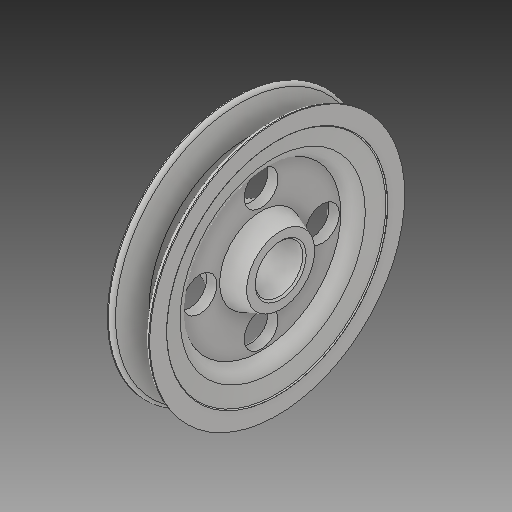
# Autodesk Inventor part: kladka
Saved by Autodesk Inventor 2019 (Build 230136000, 136)
## iProperties
Created: 2018-11-24
Part Number: kladka
Material: Generic
Document SubType Name: Modeling
Designer: Radek
Density: 1 g/cm^3
Appearance: Default
Author: Radek
Autodesk Inventor part; units mm, degrees
ref_plane "YZ Plane" through (0, 0, 0) normal (1, 0, 0) x (0, 1, 0)
ref_plane "XZ Plane" through (0, 0, 0) normal (0, 1, 0) x (-1, 0, 0)
ref_plane "XY Plane" through (0, 0, 0) normal (0, 0, 1) x (1, 0, 0)
sketch "Náčrt1" plane through (0, 0, 0) normal (0, 1, 0) x (-1, 0, 0)
  line L0 (14.5, -14) -> (-14.5, -14)
  line L1 (-14.5, -14) -> (-14.5, -20)
  line L2 (-14.5, -20) -> (-3, -24.4144)
  line L3 (-3, -24.4144) -> (-3, -46.8905)
  line L4 (14.5, -14) -> (14.5, -20)
  line L5 (14.5, -20) -> (3, -24.4144)
  line L6 (3, -24.4144) -> (3, -46.8905)
  line L7 (0, 0) -> (-43.8955, 0)
  line L8 (0, -90.4918) -> (0, 15.082) projected
  line L9 (-12.5, -75) -> (-12.5, -65)
  line L10 (12.5, -75) -> (12.5, -65)
  arc A0 (5.3126, -57.5064) -> (-5.3126, -57.5064) centre (0, -58.9299) ccw
  line L11 (-12.5, -75) -> (-11.9183, -75)
  line L12 (-9.5035, -73.147) -> (-5.3126, -57.5064)
  arc A1 (-11.9183, -75) -> (-9.5035, -73.147) centre (-11.9183, -72.5) ccw
  line L13 (12.5, -75) -> (11.9183, -75)
  line L14 (9.5035, -73.147) -> (5.3126, -57.5064)
  arc A2 (9.5035, -73.147) -> (11.9183, -75) centre (11.9183, -72.5) ccw
  line L15 (-12.5, -65) -> (-12.3924, -65)
  line L16 (-11.804, -64.517) -> (-9.808, -54.4795)
  arc A3 (-12.3924, -65) -> (-11.804, -64.517) centre (-12.3924, -64.4) ccw
  line L17 (12.5, -65) -> (12.3924, -65)
  line L18 (11.804, -64.517) -> (9.808, -54.4795)
  arc A4 (11.804, -64.517) -> (12.3924, -65) centre (12.3924, -64.4) ccw
  arc A5 (9.808, -54.4795) -> (3, -46.8905) centre (0, -56.4299) ccw
  arc A6 (-3, -46.8905) -> (-9.808, -54.4795) centre (0, -56.4299) ccw
  point P0 (-10, -75)
  point P1 (10, -75)
  point P2 (-11.9, -65)
  point P3 (11.9, -65)
  dimension "d0" = 111
  dimension "d1" = 111
  dimension "d2" = 29
  dimension "d3" = 28
  dimension "d4" = 40
  dimension "d5" = 6
  dimension "d14" = 10
  dimension "d20" = 11
  dimension "d22" = 25
  dimension "d26" = 2.5
  dimension "d27" = 15
  dimension "d28" = 2.5
  dimension "d29" = 2.5
  dimension "d30" = 2.5
  dimension "d32" = 2.5
  dimension "d33" = 0.6
  dimension "d34" = 0.6
  dimension "d35" = 0.6
  dimension "d36" = 0.6
  dimension "d37" = 3
  dimension "d38" = 150
  dimension "d39" = 11.247
  dimension "d40" = 11.247
  constraints: 36 end point, 14 point on circle, 12 tangent, 10 point on line, 7 centre point, 6 horizontal, 2 equal length, 2 parallel, 2 symmetric about line, 2 vertical, 1 perpendicular
  measures "d0" angle of L2 L3
  measures "d1" angle of L6 L5
  measures "d2" distance of L0.start L0.end
  measures "d3" diameter of L0 L7
  measures "d4" diameter of L1.end L7
  measures "d5" distance between parallel lines of L3 L6
  measures "d14" distance of L9.start L9.end
  measures "d20" diameter of A0
  measures "d22" distance between parallel lines of L9 L10
  measures "d26" distance of L9.start point (-10, -75)
  measures "d27" angle of L8 L12
  measures "d28" radius of A1
  measures "d29" distance of L10.start point (10, -75)
  measures "d30" radius of A2
  measures "d32" distance of A0.centre A5.centre
  measures "d33" distance of L9.end point (-11.9, -65)
  measures "d34" radius of A3
  measures "d35" distance of L10.end point (11.9, -65)
  measures "d36" radius of A4
  measures "d37" distance from line of A5.centre L3
  measures "d38" diameter of L9.start L7
  measures "d39" angle of L3 L16
  measures "d40" angle of L8 L18
revolve "Rotace1" add sketch "Náčrt1" angle 360 about axis through (0, 0, 0) along (1, 0, 0)
sketch "Náčrt2" plane through (0, 0, 0) normal (1, 0, 0) x (0, 1, 0)
  line L0 (-105, 0) -> (105, 0) projected
  line L1 (0, 105) -> (0, -105) projected
  circle A0 centre (0, -36) radius 10
  circle A1 centre (-36, 0) radius 10
  circle A2 centre (0, 36) radius 10
  circle A3 centre (36, 0) radius 10
  point P0 (0, 0)
  dimension "d42" = 72
  dimension "d43" = 72
  dimension "d44" = 36
  dimension "d45" = 0
  dimension "d46" = 0
  dimension "d47" = 36
  dimension "d48" = 0
  dimension "d49" = 0
  dimension "d50" = 20
  dimension "d51" = 20
  dimension "d52" = 20
  dimension "d53" = 20
  constraints: 4 centre point, 4 coincident
  measures "d42" distance of point (0, 36) point (0, -36)
  measures "d43" distance of point (36, 0) point (-36, 0)
  measures "d44" distance from line of L1 point (-36, 0)
  measures "d45" distance from line of L0 point (-36, 0)
  measures "d46" distance from line of L0 point (36, 0)
  measures "d47" distance from line of L0 point (0, 36)
  measures "d48" distance from line of L1 point (0, 36)
  measures "d49" distance from line of L1 point (0, -36)
  measures "d50" diameter of A0
  measures "d51" diameter of A1
  measures "d52" diameter of A2
  measures "d53" diameter of A3
extrude "Vysunutí1" cut sketch "Náčrt2" along normal through all both and the other way through all
chamfer "Zkosení1" distance 1 angle 45 2 edges at (14.5, 0, 14) (-14.5, 0, 14)
equation "\"d44\" = 0.5 * d43"
equation "\"d47\" = 0.5 * d42"
